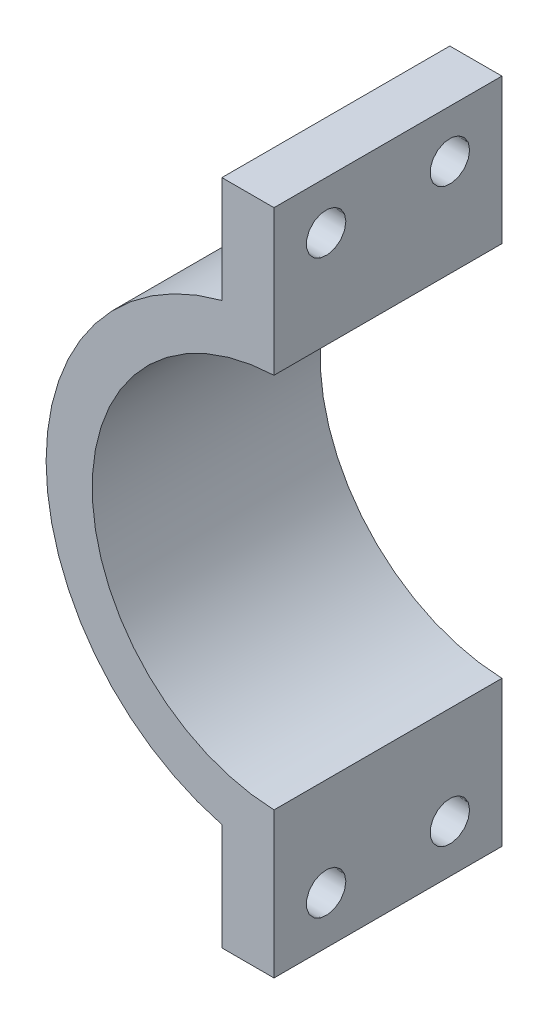
# Autodesk Inventor part: motor mount cap
Saved by Autodesk Inventor 2020 (Build 240168000, 168)
## iProperties
Created: 2019-10-28
Part Number: motor mount cap
Material: Generic
Document SubType Name: Modeling
Designer: ball
Density: 1 g/cm^3
Appearance: Default
Author: ball
Autodesk Inventor part; units mm, degrees
ref_plane "YZ Plane" through (0, 0, 0) normal (1, 0, 0) x (0, 1, 0)
ref_plane "XZ Plane" through (0, 0, 0) normal (0, 1, 0) x (-1, 0, 0)
ref_plane "XY Plane" through (0, 0, 0) normal (0, 0, 1) x (1, 0, 0)
ref_plane "Work Plane1" through (0, 0, 0) normal (0, 0, 1) x (1, 0, 0)
sketch "Sketch1" plane through (0, 0, 0) normal (0, 0, 1) x (1, 0, 0)
  arc A0 (18.9992, 41.108) -> (0, 60.0877) centre (-0.0008, 41.0877) ccw projected
  arc A1 (0, 22.1284) -> (18.9992, 41.108) centre (-0.0008, 41.1284) ccw projected
  arc A2 (44.3468, 60.0877) -> (25.3476, 41.108) centre (44.3476, 41.0877) ccw projected
  arc A3 (25.3476, 41.108) -> (44.3468, 22.1284) centre (44.3476, 41.1284) ccw projected
  arc A4 (25.3771, 40.0696) -> (25.3781, 42.1637) centre (-0.0008, 41.1284) ccw
  line L0 (-0.635, 63.9796) -> (-0.635, 59.4824)
  line L1 (-0.635, 22.7743) -> (-0.635, 18.2772)
  line L2 (10.16, 73.6386) -> (5.7912, 73.6386) construction
  line L3 (0, 77.677) -> (0, 67.7202) construction
  line L4 (5.7912, 73.6386) -> (-2.3188, 73.6386)
  line L5 (5.7912, 73.6386) -> (13.9012, 73.6386) construction
  line L6 (-25.35, 77.677) -> (-25.35, 84.027) projected
  line L7 (-25.35, -6.35) -> (-25.35, 0) projected
  line L8 (-25.35, 77.677) -> (-25.35, 0) construction
  arc A5 (-5.715, 63.2627) -> (-5.715, 18.9941) centre (-0.0008, 41.1284) ccw
  arc A6 (-5.715, 63.2627) -> (-5.715, 18.9941) centre (-0.0008, 41.1284) ccw
  line L9 (0, 66.5284) -> (0, 59.4934)
  arc A7 (-0.635, 59.4824) -> (-0.635, 22.7743) centre (-0.0008, 41.1284) ccw
  line L10 (0, 22.7634) -> (0, 16.3626)
  line L11 (-5.715, 63.2627) -> (-5.715, 73.6386)
  line L12 (-5.715, 73.6386) -> (-0.635, 73.6386)
  line L13 (-0.635, 73.6386) -> (-0.635, 63.9796)
  line L14 (10.16, 8.5775) -> (5.7912, 8.5775) construction
  line L15 (-5.715, 8.5775) -> (-0.635, 8.5775)
  line L16 (-0.635, 8.5775) -> (-0.635, 18.2772)
  line L17 (-5.715, 8.5775) -> (-5.715, 18.9941)
  point P0 (0, 0)
  point P1 (-0.635, 73.6386)
  dimension "d1" = 180
  dimension "d3" = 0.635
  dimension "d4" = 5.08
  dimension "d5" = 5.08
  constraints: 26 end point, 11 point on circle, 4 centre point, 4 vertical, 3 coincident, 2 point on line, 1 collinear, 1 horizontal, 1 parallel
  measures "d1" angle of L4 L5
  measures "d3" distance between parallel lines of L0 L9
  measures "d4" distance of L11.end L12.end
  measures "d5" distance of L15.end L15.start
ref_plane "Work Plane2" through (0, 17.6708, -22.228) normal (0, 0, -1) x (0, 1, 0)
extrude "Extrusion1" add sketch "Sketch1" against normal up to surface (22.228 mm away) contours L0 A7 L1 L16 L15 L17 A5 L11 L12 L4 L13
sketch "Sketch2" plane through (-5.715, 63.2627, 0) normal (-1, 0, 0) x (0, 0, 1)
  circle A0 centre (-17.148, 5.715) radius 1.9304
  circle A1 centre (-5.08, 5.715) radius 1.9304
  circle A2 centre (-5.08, -50.0243) radius 1.9304
  circle A3 centre (-17.148, -50.0243) radius 1.9304
  point P0 (0, -63.2627)
  constraints: 4 centre point, 8 other
extrude "Extrusion2" cut sketch "Sketch2" along normal mid plane 25.4
body "Solid1"
